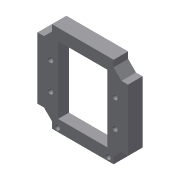
# Autodesk Inventor part: 20_Cube_Insert_RaspiCam_v3
Saved by Autodesk Inventor 2019.4 (Build 234330000, 330)
## iProperties
Created: 2019-07-01
Part Number: 20_Cube_Insert_RaspiCam_v3
Material: Generic
Document SubType Name: Modeling
Designer: diederichbenedict
Density: 1 g/cm^3
Appearance: Default
Author: diederichbenedict
Autodesk Inventor part; units mm, degrees
ref_plane "YZ Plane" through (0, 0, 0) normal (1, 0, 0) x (0, 1, 0)
ref_plane "XZ Plane" through (0, 0, 0) normal (0, 1, 0) x (-1, 0, 0)
ref_plane "Work Plane1" through (0, 0, 10) normal (0, 0, 1) x (1, 0, 0)
sketch "Sketch1" plane through (0, 0, 10) normal (0, 0, 1) x (1, 0, 0)
  line L0 (-4.0299, -0.3538) -> (-2.2322, 1.4439) construction
  arc A0 (-1.4439, 2.2322) -> (-2.2322, 1.4439) centre (-0.9299, 0.9299) ccw construction
  line L1 (-1.4439, 2.2322) -> (0.3538, 4.0299) construction
  line L2 (-37.8299, 42.2137) -> (-37.8299, 45.8299) construction
  line L3 (-37.8299, 45.8299) -> (-4.0299, 45.8299) construction
  line L4 (-4.0299, 45.8299) -> (-4.0299, 42.2137) construction
  line L5 (-4.0299, 4.0299) -> (0.3538, 4.0299) projected
  circle A1 centre (-20.9299, 20.9299) radius 17.5 construction
  line L6 (-20.9299, 58.9723) -> (17.1124, 20.9299) construction
  line L7 (17.1124, 20.9299) -> (-20.9299, -17.1124) construction
  line L8 (-20.9299, -17.1124) -> (-58.9723, 20.9299) construction
  line L9 (-58.9723, 20.9299) -> (-20.9299, 58.9723) construction
  line L10 (-20.9299, 58.9723) -> (-20.9299, -17.1124) construction
  line L11 (17.1124, 20.9299) -> (-58.9723, 20.9299) construction
  line L12 (-20.9299, 58.9723) -> (32.8701, 58.9723) construction
  line L13 (-43.2198, 43.4299) -> (1.7802, 43.4299) construction
  line L14 (1.7802, 43.4299) -> (1.7802, -1.5701) construction
  line L15 (1.7802, -1.5701) -> (-43.2198, -1.5701) construction
  line L16 (-43.2198, -1.5701) -> (-43.2198, 43.4299) construction
  line L17 (-43.2198, 5.1774) -> (-43.2198, 36.6824)
  line L18 (-43.2198, 36.6824) -> (-36.4723, 43.4299)
  line L19 (-36.4723, 43.4299) -> (-5.3876, 43.4299)
  line L20 (-5.3876, 43.4299) -> (1.7802, 36.2621)
  line L21 (1.7802, 36.2621) -> (1.7802, 5.5977)
  line L22 (1.7802, 5.5977) -> (-5.3876, -1.5701)
  line L23 (-5.3876, -1.5701) -> (-36.4723, -1.5701)
  line L24 (-36.4723, -1.5701) -> (-43.2198, 5.1774)
  line L25 (-4.0299, 42.2137) -> (-37.8299, 42.2137) projected
  line L26 (-4.0299, -0.3538) -> (-4.0299, 4.0299) projected
  line L27 (-43.2198, 43.4299) -> (-10.4667, 10.6769) construction
  line L28 (-8.5595, 8.5517) -> (1.7802, -1.5701) construction
  line L29 (1.7802, 43.4299) -> (-25.699, 15.9507) construction
  line L30 (-30.9728, 10.6769) -> (-43.2198, -1.5701) construction
  point P0 (-37.8299, 4.0299)
  dimension "d18" = 53.8
  dimension "d19" = 45
  dimension "d20" = 53.8
  dimension "d21" = 45
  dimension "d22" = 45
  constraints: 46 end point, 15 point on line, 4 parallel, 3 perpendicular, 2 horizontal, 2 midpoint, 1 equal length, 2 other
  measures "d18" distance of L6.start L6.end
  measures "d19" angle of L6 L12
  measures "d20" distance of L6.end L7.end
  measures "d21" distance of L14.end L15.end
  measures "d22" distance of L13.end L14.end
extrude "Extrusion1" add sketch "Sketch1" along normal blind 8
sketch "Sketch3" plane through (0, 0, 10) normal (0, 0, -1) x (-1, 0, 0)
  line L0 (37.8299, -0.4701) -> (37.8299, 4.0299) construction
  line L1 (4.0299, 4.0299) -> (4.0299, -0.4701) construction
  line L2 (37.8299, -0.4701) -> (37.8299, 1.1886) construction
  line L3 (4.0299, -3.9701) -> (4.0299, -0.3538) construction
  line L4 (45.8299, 4.0299) -> (42.2137, 4.0299) construction
  line L5 (-0.3538, 4.0299) -> (-3.9701, 4.0299) construction
  line L6 (-3.9701, 37.8299) -> (-0.3538, 37.8299) construction
  line L7 (4.0299, 42.2137) -> (4.0299, 45.8299) construction
  line L8 (37.8299, 45.8299) -> (37.8299, 42.2137) construction
  line L9 (42.2137, 37.8299) -> (45.8299, 37.8299) construction
  line L10 (37.8299, 37.7299) -> (45.8299, 37.7299)
  line L11 (45.8299, 37.7299) -> (45.8299, 4.1299)
  line L12 (45.8299, 4.1299) -> (37.8299, 4.1299)
  line L13 (37.8299, 4.1299) -> (37.8299, 37.7299)
  line L14 (37.7299, 4.0299) -> (4.1299, 4.0299)
  line L15 (4.1299, 4.0299) -> (4.1299, -3.9701)
  line L16 (4.1299, -3.9701) -> (37.7299, -3.9701)
  line L17 (37.7299, -3.9701) -> (37.7299, 4.0299)
  line L18 (4.0299, 4.1299) -> (-3.9701, 4.1299)
  line L19 (-3.9701, 4.1299) -> (-3.9701, 37.7299)
  line L20 (-3.9701, 37.7299) -> (4.0299, 37.7299)
  line L21 (4.0299, 37.7299) -> (4.0299, 4.1299)
  line L22 (4.1299, 37.8299) -> (37.7299, 37.8299)
  line L23 (37.7299, 37.8299) -> (37.7299, 45.8299)
  line L24 (37.7299, 45.8299) -> (4.1299, 45.8299)
  line L25 (4.1299, 45.8299) -> (4.1299, 37.8299)
  point P0 (0, 0)
  dimension "d23" = 0.1
  dimension "d24" = 0.1
  dimension "d25" = 0.1
  dimension "d26" = 0.1
  dimension "d27" = 0.1
  constraints: 32 end point, 8 parallel, 4 horizontal, 4 perpendicular, 3 point on line
  measures "d23" distance between parallel lines of L8 L23
  measures "d24" distance between parallel lines of L7 L25
  measures "d25" distance between parallel lines of L6 L20
  measures "d26" distance between parallel lines of L5 L18
  measures "d27" distance between parallel lines of L1 L15
extrude "Extrusion3" add sketch "Sketch3" against normal up to surface (8 mm away)
sketch "Skizze12" plane through (0, 0, 10) normal (0, 0, -1) x (-1, 0, 0)
  line L0 (-0.3124, 4.1299) -> (4.1299, -0.3124) projected
  line L1 (4.1299, -0.3124) -> (4.1299, -3.9701) projected
  line L2 (4.1299, -3.9701) -> (37.7299, -3.9701) construction
  line L3 (37.7299, -3.9701) -> (37.7299, -0.3124) projected
  line L4 (37.7299, -0.3124) -> (42.1723, 4.1299) projected
  line L5 (45.8299, 4.1299) -> (42.1723, 4.1299) projected
  line L6 (45.8299, 37.7299) -> (45.8299, 4.1299) construction
  line L7 (42.1723, 37.7299) -> (45.8299, 37.7299) projected
  line L8 (42.1723, 37.7299) -> (37.7299, 42.1723) projected
  line L9 (37.7299, 42.1723) -> (37.7299, 45.8299) projected
  line L10 (37.7299, 45.8299) -> (4.1299, 45.8299) construction
  line L11 (4.1299, 45.8299) -> (4.1299, 42.1723) projected
  line L12 (4.1299, 42.1723) -> (-0.3124, 37.7299) projected
  line L13 (-3.9701, 37.7299) -> (-0.3124, 37.7299) projected
  line L14 (-3.9701, 4.1299) -> (-3.9701, 37.7299) construction
  line L15 (-0.3124, 4.1299) -> (-3.9701, 4.1299) projected
  line L16 (37.9299, -4.1701) -> (3.9299, -4.1701) construction
  line L17 (3.9299, -4.1701) -> (3.9299, -0.3953)
  line L18 (3.9299, -0.3953) -> (-0.3953, 3.9299)
  line L19 (-0.3953, 3.9299) -> (-4.1701, 3.9299)
  line L20 (-4.1701, 3.9299) -> (-4.1701, 37.9299) construction
  line L21 (-4.1701, 37.9299) -> (-0.3953, 37.9299)
  line L22 (-0.3953, 37.9299) -> (3.9299, 42.2551)
  line L23 (3.9299, 42.2551) -> (3.9299, 46.0299)
  line L24 (3.9299, 46.0299) -> (37.9299, 46.0299) construction
  line L25 (37.9299, 46.0299) -> (37.9299, 42.2551)
  line L26 (37.9299, 42.2551) -> (42.2551, 37.9299)
  line L27 (42.2551, 37.9299) -> (46.0299, 37.9299)
  line L28 (46.0299, 37.9299) -> (46.0299, 3.9299) construction
  line L29 (46.0299, 3.9299) -> (42.2551, 3.9299)
  line L30 (42.2551, 3.9299) -> (37.9299, -0.3953)
  line L31 (37.9299, -0.3953) -> (37.9299, -4.1701)
  line L32 (-3.9701, 37.7299) -> (-3.9701, 37.9299)
  line L33 (37.7299, 45.8299) -> (4.1299, 45.8299) projected
  line L34 (4.1299, 45.8299) -> (3.9299, 45.8299)
  line L35 (37.7299, 45.8299) -> (37.9299, 45.8299)
  line L36 (45.8299, 37.7299) -> (45.8299, 37.9299)
  line L37 (45.8299, 4.1299) -> (45.8299, 3.9299)
  line L38 (37.7299, -3.9701) -> (37.9299, -3.9701)
  line L39 (4.1299, -3.9701) -> (3.9299, -3.9701)
  line L40 (-3.9701, 4.1299) -> (-3.9701, 3.9299)
  point P0 (0, 0)
  dimension "d65" = 0.2
  constraints: 48 end point, 13 point on line, 2 perpendicular, 1 vertical, 15 other
  measures "d65" distance between parallel lines of L2 L16
extrude "IM_offset" add sketch "Skizze12" against normal up to surface (8 mm away)
sketch "Sketch15" plane through (0, 0, 10) normal (0, 0, -1) x (-1, 0, 0)
  line L0 (-3.9701, 3.9299) -> (-3.9701, 37.9299) projected
  line L1 (-0.3953, 3.9299) -> (-3.9701, 3.9299) projected
  line L2 (3.9299, -0.3953) -> (-0.3953, 3.9299) projected
  line L3 (3.9299, -3.9701) -> (3.9299, -0.3953) projected
  line L4 (3.9299, -3.9701) -> (37.9299, -3.9701) projected
  line L5 (37.9299, -0.3953) -> (37.9299, -3.9701) projected
  line L6 (42.2551, 3.9299) -> (37.9299, -0.3953) projected
  line L7 (45.8299, 3.9299) -> (42.2551, 3.9299) projected
  line L8 (45.8299, 3.9299) -> (45.8299, 37.9299) projected
  line L9 (45.8299, 37.9299) -> (42.2551, 37.9299) projected
  line L10 (42.2551, 37.9299) -> (37.9299, 42.2551) projected
  line L11 (37.9299, 42.2551) -> (37.9299, 45.8299) projected
  line L12 (37.9299, 45.8299) -> (3.9299, 45.8299) projected
  line L13 (3.9299, 45.8299) -> (3.9299, 42.2551) projected
  line L14 (3.9299, 42.2551) -> (-0.3953, 37.9299) projected
  line L15 (-0.3953, 37.9299) -> (-3.9701, 37.9299) projected
  line L16 (37.4799, 42.3799) -> (4.4799, 42.3799)
  line L17 (4.4799, 42.3799) -> (4.4799, -0.6201)
  line L18 (4.4799, -0.6201) -> (37.4799, -0.6201)
  line L19 (37.4799, -0.6201) -> (37.4799, 42.3799)
  line L20 (37.4799, 42.3799) -> (4.4799, -0.6201) construction
  line L21 (4.4799, 42.3799) -> (37.4799, -0.6201) construction
  circle A0 centre (20.9799, 20.8799) radius 16.97 construction
  point P0 (0, 0)
  dimension "d73" = 33
  dimension "d74" = 43
  dimension "d90" = 21.5
  dimension "d91" = 16.5
  constraints: 12 end point, 2 midpoint, 2 parallel, 1 horizontal, 1 perpendicular
  measures "d73" distance of L18.end L17.end
  measures "d74" distance of L17.end L16.end
  measures "d90" distance from line of A0.centre L16
  measures "d91" distance from line of A0.centre L17
extrude "Extrusion13" cut sketch "Sketch15" against normal blind 2 contours L19 L18 L17 L16
sketch "Sketch16" plane through (0, 0, 12) normal (0, 0, -1) x (-1, 0, 0)
  line L0 (4.4799, 42.3799) -> (37.4799, 42.3799) projected
  line L1 (4.4799, -0.6201) -> (4.4799, 42.3799) projected
  line L2 (37.4799, -0.6201) -> (4.4799, -0.6201) projected
  line L3 (37.4799, 42.3799) -> (37.4799, -0.6201) projected
  line L4 (7.4799, 39.3799) -> (34.4799, 39.3799)
  line L5 (34.4799, 39.3799) -> (34.4799, 2.3799)
  line L6 (34.4799, 2.3799) -> (7.4799, 2.3799)
  line L7 (7.4799, 2.3799) -> (7.4799, 39.3799)
  dimension "d94" = 3
  constraints: 8 end point, 3 other
  measures "d94" distance between parallel lines of L1 L7
extrude "Extrusion14" cut sketch "Sketch16" against normal through all contours L4 L5 L6 L7
sketch "Sketch17" plane through (0, 0, 10) normal (0, 0, -1) x (-1, 0, 0)
  line L0 (37.4799, 42.3799) -> (37.4799, -0.6201) projected
  line L1 (4.4799, -0.6201) -> (4.4799, 42.3799) projected
  line L2 (38.7299, 28.3799) -> (3.2299, 28.3799)
  line L3 (3.2299, 28.3799) -> (3.2299, 13.3799)
  line L4 (3.2299, 13.3799) -> (38.7299, 13.3799)
  line L5 (38.7299, 13.3799) -> (38.7299, 28.3799)
  line L6 (38.7299, 28.3799) -> (3.2299, 13.3799) construction
  line L7 (3.2299, 28.3799) -> (38.7299, 13.3799) construction
  line L8 (4.4799, 42.3799) -> (37.4799, 42.3799) projected
  circle A0 centre (20.9799, 20.8799) radius 16.97 construction
  line L9 (37.4799, -0.6201) -> (4.4799, -0.6201) projected
  point P0 (0, 0)
  dimension "d81" = 35.5
  dimension "d82" = 15
  dimension "d92" = 0
  dimension "d93" = 0
  constraints: 12 end point, 2 midpoint, 2 parallel, 1 horizontal, 1 perpendicular
  measures "d81" distance of L4.end L3.end
  measures "d82" distance of L3.end L2.end
  measures "d92" distance of A0.centre point (20.98, 20.88)
  measures "d93" distance of A0.centre point (20.98, 20.88)
hole "Hole1" at (-3.2299, 13.3799, 10) at (-3.2299, 28.3799, 10) at (-38.7299, 28.3799, 10) at (-38.7299, 13.3799, 10) direction (0, 0, 1) diameter 2.8 end through all
sketch "Sketch18" plane through (0, 0, 10) normal (0, 0, -1) x (-1, 0, 0)
  line L0 (45.3299, 43.7299) -> (45.3299, -1.9701) projected
  line L1 (37.9499, -0.2701) -> (37.9499, -3.9701) projected
  line L2 (4.0099, -3.9701) -> (4.0099, 0.1299) projected
  circle A0 centre (6.9799, -1.9201) radius 1.4
  circle A1 centre (34.9799, -1.9201) radius 1.4
  circle A2 centre (20.9799, 20.8799) radius 16.97 construction
  circle A3 centre (20.9799, 20.8799) radius 16.97 construction
  point P0 (0, 0)
  dimension "d95" = 2.8
  dimension "d96" = 2.8
  dimension "d97" = 14
  dimension "d98" = 14
  constraints: 2 centre point
  measures "d95" diameter of A0
  measures "d96" diameter of A1
  measures "d97" horizontal distance of A0.centre A2.centre
  measures "d98" horizontal distance of A1.centre A2.centre
extrude "Extrusion15" cut sketch "Sketch18" against normal blind 10
body "Solid1"
